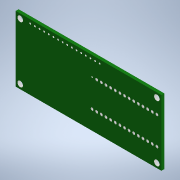
# Autodesk Inventor part: PCB
Saved by Autodesk Inventor 2020.1 (Build 241239000, 239)
## iProperties
Created: 2019-12-09
Part Number: PCB
Material: Generic
Document SubType Name: Modeling
Designer: Daniel
Density: 1 g/cm^3
Appearance: Default
Author: Daniel
Autodesk Inventor part; units mm, degrees
ref_plane "YZ Plane" through (0, 0, 0) normal (1, 0, 0) x (0, 1, 0)
ref_plane "XZ Plane" through (0, 0, 0) normal (0, 1, 0) x (-1, 0, 0)
ref_plane "XY Plane" through (0, 0, 0) normal (0, 0, 1) x (1, 0, 0)
sketch "Sketch1" plane through (0, 0, 0) normal (0, 0, 1) x (1, 0, 0)
  line L0 (-40, -18) -> (40, -18)
  line L1 (40, -18) -> (40, 18)
  line L2 (40, 18) -> (-40, 18)
  line L3 (-40, 18) -> (-40, -18)
  line L4 (-40, -18) -> (40, 18) construction
  line L5 (40, -18) -> (-40, 18) construction
  point P0 (0, 0)
  dimension "d0" = 36
  dimension "d1" = 80
  constraints: 12 end point, 2 midpoint, 2 parallel, 1 horizontal, 1 perpendicular
  measures "d0" distance of L0.end L1.end
  measures "d1" distance of L1.end L2.end
extrude "Extrusion1" add sketch "Sketch1" along normal blind 1.6
sketch "Sketch2" plane through (0, 0, 1.6) normal (0, 0, 1) x (1, 0, 0)
  line L0 (-37.5, -15.5) -> (37.5, -15.5) construction
  line L1 (37.5, -15.5) -> (37.5, 15.5) construction
  line L2 (37.5, 15.5) -> (-37.5, 15.5) construction
  line L3 (-37.5, 15.5) -> (-37.5, -15.5) construction
  line L4 (-37.5, -15.5) -> (37.5, 15.5) construction
  line L5 (37.5, -15.5) -> (-37.5, 15.5) construction
  point P0 (0, 0)
  dimension "d4" = 31
  dimension "d5" = 75
  constraints: 12 end point, 4 coincident, 2 midpoint, 2 parallel, 1 horizontal, 1 perpendicular
  measures "d4" distance of L0.end L1.end
  measures "d5" distance of L1.end L2.end
hole "Hole1" at (-37.5, 15.5, 1.6) at (37.5, 15.5, 1.6) at (37.5, -15.5, 1.6) at (-37.5, -15.5, 1.6) direction (0, 0, -1) diameter 3 depth 10 tip angle 118
sketch "Sketch3" plane through (0, 0, 0) normal (0, 0, -1) x (-1, 0, 0)
  line L0 (27.245, 16.325) -> (27.245, 15.675)
  line L1 (27.245, 15.675) -> (26.595, 15.675)
  line L2 (26.595, 15.675) -> (26.595, 16.325)
  line L3 (26.595, 16.325) -> (27.245, 16.325)
  line L4 (24.705, 16.325) -> (24.705, 15.675)
  line L5 (24.705, 15.675) -> (24.055, 15.675)
  line L6 (24.055, 15.675) -> (24.055, 16.325)
  line L7 (24.055, 16.325) -> (24.705, 16.325)
  line L8 (22.165, 16.325) -> (22.165, 15.675)
  line L9 (22.165, 15.675) -> (21.515, 15.675)
  line L10 (21.515, 15.675) -> (21.515, 16.325)
  line L11 (21.515, 16.325) -> (22.165, 16.325)
  line L12 (19.625, 16.325) -> (19.625, 15.675)
  line L13 (19.625, 15.675) -> (18.975, 15.675)
  line L14 (18.975, 15.675) -> (18.975, 16.325)
  line L15 (18.975, 16.325) -> (19.625, 16.325)
  line L16 (17.085, 16.325) -> (17.085, 15.675)
  line L17 (17.085, 15.675) -> (16.435, 15.675)
  line L18 (16.435, 15.675) -> (16.435, 16.325)
  line L19 (16.435, 16.325) -> (17.085, 16.325)
  line L20 (14.545, 16.325) -> (14.545, 15.675)
  line L21 (14.545, 15.675) -> (13.895, 15.675)
  line L22 (13.895, 15.675) -> (13.895, 16.325)
  line L23 (13.895, 16.325) -> (14.545, 16.325)
  line L24 (4.385, 16.325) -> (4.385, 15.675)
  line L25 (4.385, 15.675) -> (3.735, 15.675)
  line L26 (3.735, 15.675) -> (3.735, 16.325)
  line L27 (3.735, 16.325) -> (4.385, 16.325)
  line L28 (1.845, 16.325) -> (1.845, 15.675)
  line L29 (1.845, 15.675) -> (1.195, 15.675)
  line L30 (1.195, 15.675) -> (1.195, 16.325)
  line L31 (1.195, 16.325) -> (1.845, 16.325)
  line L32 (-0.695, 16.325) -> (-0.695, 15.675)
  line L33 (-0.695, 15.675) -> (-1.345, 15.675)
  line L34 (-1.345, 15.675) -> (-1.345, 16.325)
  line L35 (-1.345, 16.325) -> (-0.695, 16.325)
  line L36 (-3.235, 16.325) -> (-3.235, 15.675)
  line L37 (-3.235, 15.675) -> (-3.885, 15.675)
  line L38 (-3.885, 15.675) -> (-3.885, 16.325)
  line L39 (-3.885, 16.325) -> (-3.235, 16.325)
  line L40 (-5.775, 16.325) -> (-5.775, 15.675)
  line L41 (-5.775, 15.675) -> (-6.425, 15.675)
  line L42 (-6.425, 15.675) -> (-6.425, 16.325)
  line L43 (-6.425, 16.325) -> (-5.775, 16.325)
  line L44 (29.785, 16.325) -> (29.785, 15.675)
  line L45 (29.785, 15.675) -> (29.135, 15.675)
  line L46 (29.135, 15.675) -> (29.135, 16.325)
  line L47 (29.135, 16.325) -> (29.785, 16.325)
  line L48 (12.005, 16.325) -> (12.005, 15.675)
  line L49 (12.005, 15.675) -> (11.355, 15.675)
  line L50 (11.355, 15.675) -> (11.355, 16.325)
  line L51 (11.355, 16.325) -> (12.005, 16.325)
  line L52 (9.465, 16.325) -> (9.465, 15.675)
  line L53 (9.465, 15.675) -> (8.815, 15.675)
  line L54 (8.815, 15.675) -> (8.815, 16.325)
  line L55 (8.815, 16.325) -> (9.465, 16.325)
  line L56 (6.925, 16.325) -> (6.925, 15.675)
  line L57 (6.925, 15.675) -> (6.275, 15.675)
  line L58 (6.275, 15.675) -> (6.275, 16.325)
  line L59 (6.275, 16.325) -> (6.925, 16.325)
  line L60 (32.325, 16.325) -> (32.325, 15.675)
  line L61 (32.325, 15.675) -> (31.675, 15.675)
  line L62 (31.675, 15.675) -> (31.675, 16.325)
  line L63 (31.675, 16.325) -> (32.325, 16.325)
  circle A0 centre (-6.1, 16) radius 0.75
  line L64 (-6.425, 16.325) -> (-5.775, 15.675) construction
  circle A1 centre (-6.1, 16) radius 0.4596
  circle A2 centre (-3.56, 16) radius 0.75
  circle A3 centre (-3.56, 16) radius 0.4596
  circle A4 centre (-1.02, 16) radius 0.75
  circle A5 centre (-1.02, 16) radius 0.4596
  circle A6 centre (1.52, 16) radius 0.75
  circle A7 centre (1.52, 16) radius 0.4596
  circle A8 centre (4.06, 16) radius 0.75
  circle A9 centre (4.06, 16) radius 0.4596
  circle A10 centre (6.6, 16) radius 0.75
  circle A11 centre (6.6, 16) radius 0.4596
  circle A12 centre (9.14, 16) radius 0.75
  circle A13 centre (9.14, 16) radius 0.4596
  circle A14 centre (11.68, 16) radius 0.75
  circle A15 centre (11.68, 16) radius 0.4596
  circle A16 centre (14.22, 16) radius 0.75
  circle A17 centre (14.22, 16) radius 0.4596
  circle A18 centre (16.76, 16) radius 0.75
  circle A19 centre (16.76, 16) radius 0.4596
  circle A20 centre (19.3, 16) radius 0.75
  circle A21 centre (19.3, 16) radius 0.4596
  circle A22 centre (21.84, 16) radius 0.75
  circle A23 centre (21.84, 16) radius 0.4596
  circle A24 centre (24.38, 16) radius 0.75
  circle A25 centre (24.38, 16) radius 0.4596
  circle A26 centre (26.92, 16) radius 0.75
  circle A27 centre (26.92, 16) radius 0.4596
  circle A28 centre (29.46, 16) radius 0.75
  circle A29 centre (29.46, 16) radius 0.4596
  circle A30 centre (32, 16) radius 0.75
  circle A31 centre (32, 16) radius 0.4596
  point P0 (0, 0)
  point P1 (-3.235, 16.325)
  point P2 (-0.695, 16.325)
  point P3 (1.845, 16.325)
  point P4 (4.385, 16.325)
  point P5 (6.925, 16.325)
  point P6 (9.465, 16.325)
  point P7 (12.005, 16.325)
  point P8 (14.545, 16.325)
  point P9 (17.085, 16.325)
  point P10 (19.625, 16.325)
  point P11 (22.165, 16.325)
  point P12 (24.705, 16.325)
  point P13 (27.245, 16.325)
  point P14 (29.785, 16.325)
  point P15 (32.325, 16.325)
  dimension "d15" = 1.5
  dimension "d18" = 2.54
  constraints: 130 end point, 48 horizontal, 32 vertical, 16 centre point, 16 coincident, 2 midpoint, 172 other
  measures "d15" diameter of A0
  measures "d18" distance of A0.centre A2.centre
extrude "Extrusion2" cut sketch "Sketch3" against normal blind 10 contours A27 L0 | L0 L1 L2 L3 | L3 A27 | A27 L1 | L2 A27 | A25 L4 | L4 L5 L6 L7 | L7 A25 | A25 L5 | L6 A25 | A23 L8 | L8 L9 L10 L11 | L11 A23 | A23 L9 | L10 A23 | A21 L12 | L12 L13 L14 L15 | L15 A21 | A21 L13 | L14 A21 | A19 L16 | L16 L17 L18 L19 | L19 A19 | A19 L17 | L18 A19 | A17 L20 | L20 L21 L22 L23 | L23 A17 | A17 L21 | L22 A17 | A9 L24 | L24 L25 L26 L27 | L27 A9 | A9 L25 | L26 A9 | A7 L28 | L28 L29 L30 L31 | L31 A7 | A7 L29 | L30 A7 | A5 L32 | L32 L33 L34 L35 | L35 A5 | A5 L33 | L34 A5 | A3 L36 | L36 L37 L38 L39 | L39 A3 | A3 L37 | L38 A3 | A1 L40 | L40 L41 L42 L43 | L43 A1 | A1 L41 | L42 A1 | A29 L44 | L44 L45 L46 L47 | L47 A29 | A29 L45 | L46 A29 | A15 L48 | L48 L49 L50 L51 | L51 A15 | A15 L49 | L50 A15 | A13 L52 | L52 L53 L54 L55 | L55 A13 | A13 L53 | L54 A13 | A11 L56 | L56 L57 L58 L59 | L59 A11 | A11 L57 | L58 A11 | A31 L60 | L60 L61 L62 L63 | L63 A31 | A31 L61 | L62 A31
extrude "Extrusion3" cut sketch "Sketch3" against normal blind 0.1 contours A27 L0 | L0 L1 L2 L3 | L3 A27 | A27 L1 | L2 A27 | A25 L4 | L4 L5 L6 L7 | L7 A25 | A25 L5 | L6 A25 | A23 L8 | L8 L9 L10 L11 | L11 A23 | A23 L9 | L10 A23 | A21 L12 | L12 L13 L14 L15 | L15 A21 | A21 L13 | L14 A21 | A19 L16 | L16 L17 L18 L19 | L19 A19 | A19 L17 | L18 A19 | A17 L20 | L20 L21 L22 L23 | L23 A17 | A17 L21 | L22 A17 | A9 L24 | L24 L25 L26 L27 | L27 A9 | A9 L25 | L26 A9 | A7 L28 | L28 L29 L30 L31 | L31 A7 | A7 L29 | L30 A7 | A5 L32 | L32 L33 L34 L35 | L35 A5 | A5 L33 | L34 A5 | A3 L36 | L36 L37 L38 L39 | L39 A3 | A3 L37 | L38 A3 | A1 L40 | L40 L41 L42 L43 | L43 A1 | A1 L41 | L42 A1 | A29 L44 | L44 L45 L46 L47 | L47 A29 | A29 L45 | L46 A29 | A15 L48 | L48 L49 L50 L51 | L51 A15 | A15 L49 | L50 A15 | A13 L52 | L52 L53 L54 L55 | L55 A13 | A13 L53 | L54 A13 | A11 L56 | L56 L57 L58 L59 | L59 A11 | A11 L57 | L58 A11 | A31 L60 | L60 L61 L62 L63 | L63 A31 | A31 L61 | L62 A31 | A0 | A2 | A4 | A6 | A8 | A10 | A12 | A14 | A16 | A18 | A20 | A22 | A24 | A26 | A28 | A30
sketch "Sketch4" plane through (0, 0, 1.6) normal (0, 0, 1) x (1, 0, 0)
  circle A0 centre (1.97, 7.53) radius 0.3816
  circle A1 centre (1.97, 7.53) radius 0.75
  line L0 (1.645, 7.73) -> (2.295, 7.73)
  line L1 (2.295, 7.73) -> (2.295, 7.33)
  line L2 (2.295, 7.33) -> (1.645, 7.33)
  line L3 (1.645, 7.33) -> (1.645, 7.73)
  line L4 (4.185, 7.73) -> (4.835, 7.73)
  line L5 (4.835, 7.73) -> (4.835, 7.33)
  line L6 (4.835, 7.33) -> (4.185, 7.33)
  line L7 (4.185, 7.33) -> (4.185, 7.73)
  line L8 (1.645, -7.51) -> (2.295, -7.51)
  line L9 (2.295, -7.51) -> (2.295, -7.91)
  line L10 (2.295, -7.91) -> (1.645, -7.91)
  line L11 (1.645, -7.91) -> (1.645, -7.51)
  line L12 (1.645, 7.73) -> (2.295, 7.33) construction
  circle A2 centre (4.51, 7.53) radius 0.3816
  circle A3 centre (4.51, 7.53) radius 0.75
  circle A4 centre (7.05, 7.53) radius 0.3816
  circle A5 centre (7.05, 7.53) radius 0.75
  circle A6 centre (9.59, 7.53) radius 0.3816
  circle A7 centre (9.59, 7.53) radius 0.75
  circle A8 centre (12.13, 7.53) radius 0.3816
  circle A9 centre (12.13, 7.53) radius 0.75
  circle A10 centre (14.67, 7.53) radius 0.3816
  circle A11 centre (14.67, 7.53) radius 0.75
  circle A12 centre (17.21, 7.53) radius 0.3816
  circle A13 centre (17.21, 7.53) radius 0.75
  circle A14 centre (19.75, 7.53) radius 0.3816
  circle A15 centre (19.75, 7.53) radius 0.75
  circle A16 centre (22.29, 7.53) radius 0.3816
  circle A17 centre (22.29, 7.53) radius 0.75
  circle A18 centre (24.83, 7.53) radius 0.3816
  circle A19 centre (24.83, 7.53) radius 0.75
  circle A20 centre (27.37, 7.53) radius 0.3816
  circle A21 centre (27.37, 7.53) radius 0.75
  circle A22 centre (29.91, 7.53) radius 0.3816
  circle A23 centre (29.91, 7.53) radius 0.75
  circle A24 centre (32.45, 7.53) radius 0.3816
  circle A25 centre (32.45, 7.53) radius 0.75
  circle A26 centre (34.99, 7.53) radius 0.3816
  circle A27 centre (34.99, 7.53) radius 0.75
  circle A28 centre (37.53, 7.53) radius 0.3816
  circle A29 centre (37.53, 7.53) radius 0.75
  circle A30 centre (1.97, -7.71) radius 0.3816
  circle A31 centre (1.97, -7.71) radius 0.75
  circle A32 centre (4.51, -7.71) radius 0.3816
  circle A33 centre (4.51, -7.71) radius 0.75
  circle A34 centre (7.05, -7.71) radius 0.3816
  circle A35 centre (7.05, -7.71) radius 0.75
  circle A36 centre (9.59, -7.71) radius 0.3816
  circle A37 centre (9.59, -7.71) radius 0.75
  circle A38 centre (12.13, -7.71) radius 0.3816
  circle A39 centre (12.13, -7.71) radius 0.75
  circle A40 centre (14.67, -7.71) radius 0.3816
  circle A41 centre (14.67, -7.71) radius 0.75
  circle A42 centre (17.21, -7.71) radius 0.3816
  circle A43 centre (17.21, -7.71) radius 0.75
  circle A44 centre (19.75, -7.71) radius 0.3816
  circle A45 centre (19.75, -7.71) radius 0.75
  circle A46 centre (22.29, -7.71) radius 0.3816
  circle A47 centre (22.29, -7.71) radius 0.75
  circle A48 centre (24.83, -7.71) radius 0.3816
  circle A49 centre (24.83, -7.71) radius 0.75
  circle A50 centre (27.37, -7.71) radius 0.3816
  circle A51 centre (27.37, -7.71) radius 0.75
  circle A52 centre (29.91, -7.71) radius 0.3816
  circle A53 centre (29.91, -7.71) radius 0.75
  circle A54 centre (32.45, -7.71) radius 0.3816
  circle A55 centre (32.45, -7.71) radius 0.75
  circle A56 centre (34.99, -7.71) radius 0.3816
  circle A57 centre (34.99, -7.71) radius 0.75
  circle A58 centre (37.53, -7.71) radius 0.3816
  circle A59 centre (37.53, -7.71) radius 0.75
  point P0 (0, 0)
  point P1 (4.835, 7.73)
  point P2 (7.375, 7.73)
  point P3 (9.915, 7.73)
  point P4 (12.455, 7.73)
  point P5 (14.995, 7.73)
  point P6 (17.535, 7.73)
  point P7 (20.075, 7.73)
  point P8 (22.615, 7.73)
  point P9 (25.155, 7.73)
  point P10 (27.695, 7.73)
  point P11 (30.235, 7.73)
  point P12 (32.775, 7.73)
  point P13 (35.315, 7.73)
  point P14 (37.855, 7.73)
  point P15 (2.295, -7.51)
  point P16 (4.835, -7.51)
  point P17 (7.375, -7.51)
  point P18 (9.915, -7.51)
  point P19 (12.455, -7.51)
  point P20 (14.995, -7.51)
  point P21 (17.535, -7.51)
  point P22 (20.075, -7.51)
  point P23 (22.615, -7.51)
  point P24 (25.155, -7.51)
  point P25 (27.695, -7.51)
  point P26 (30.235, -7.51)
  point P27 (32.775, -7.51)
  point P28 (35.315, -7.51)
  point P29 (37.855, -7.51)
  dimension "d25" = 1.5
  dimension "d40" = 2.54
  dimension "d43" = 15.24
  constraints: 30 centre point, 30 coincident, 26 end point, 22 vertical, 21 horizontal, 2 midpoint, 218 other
  measures "d25" diameter of A1
  measures "d40" distance of point (1.97, 7.53) point (4.51, 7.53)
  measures "d43" distance of point (1.97, 7.53) point (1.97, -7.71)
extrude "Extrusion4" cut sketch "Sketch4" against normal blind 10 contours A0 L1 | L0 A0 | L1 L2 L3 L0 | A0 L2 | L3 A0 | A2 L4 | L4 L5 L6 L7 | L7 A2 | A2 L5 | L6 A2 | A30 L8 | L8 L9 L10 L11 | L11 A30 | A30 L9 | L10 A30 | A4 | A6 | A8 | A10 | A12 | A14 | A16 | A18 | A20 | A22 | A24 | A26 | A28 | A32 | A34 | A36 | A38 | A40 | A42 | A44 | A46 | A48 | A50 | A52 | A54 | A56 | A58
extrude "Extrusion5" cut sketch "Sketch4" against normal blind 0.1 contours A2 L4 | L4 L5 L6 L7 | L7 A2 | A2 L5 | L6 A2 | A30 L8 | L8 L9 L10 L11 | L11 A30 | A30 L9 | L10 A30 | A3 | A4 | A5 | A6 | A7 | A8 | A9 | A10 | A11 | A12 | A13 | A14 | A15 | A16 | A17 | A18 | A19 | A20 | A21 | A22 | A23 | A24 | A25 | A26 | A27 | A28 | A29 | A31 | A32 | A33 | A34 | A35 | A36 | A37 | A38 | A39 | A40 | A41 | A42 | A43 | A44 | A45 | A46 | A47 | A48 | A49 | A50 | A51 | A52 | A53 | A54 | A55 | A56 | A57 | A58 | A59
body "Solid1"
